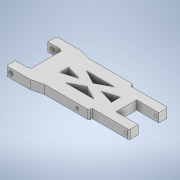
# Autodesk Inventor part: PX9200-10
Saved by Autodesk Inventor 2022.3 (Build 263350000, 350)
## iProperties
Created: 2022-07-14
Part Number: PX9200-10
Material: Generic
Document SubType Name: Modeling
Designer: luis_
Density: 1 g/cm^3
Appearance: Default
Author: luis_
Autodesk Inventor part; units mm, degrees
ref_plane "YZ Plane" through (0, 0, 0) normal (1, 0, 0) x (0, 1, 0)
ref_plane "XZ Plane" through (0, 0, 0) normal (0, 1, 0) x (-1, 0, 0)
ref_plane "XY Plane" through (0, 0, 0) normal (0, 0, 1) x (1, 0, 0)
sketch "Sketch1" plane through (0, 0, 0) normal (0, 1, 0) x (-1, 0, 0)
  line L0 (39.5, 16.9949) -> (118.5, 16.9949) construction
  line L1 (31.5, 10.9949) -> (39.5, 10.9949)
  line L2 (39.5, -11.0051) -> (31.5, -11.0051)
  line L3 (29.5, -10.0051) -> (31.5, -11.0051)
  line L4 (29.5, 9.9949) -> (31.5, 10.9949)
  line L5 (29.5, 9.9949) -> (29.5, -10.0051)
  line L6 (39.5, -17.0051) -> (39.5, -11.0051)
  line L7 (39.5, 10.9949) -> (39.5, 16.9949)
  line L8 (-14.5, 15) -> (15.5, 15)
  line L9 (15.5, -15) -> (-14.5, -15)
  line L10 (15.5, 15) -> (23.5, 16.9949)
  line L11 (15.5, -15) -> (23.5, -17.0051)
  line L12 (39.5, -17.0051) -> (23.5, -17.0051)
  line L13 (39.5, 16.9949) -> (23.5, 16.9949)
  line L14 (-39.5, 13) -> (-14.5, 13)
  line L15 (-39.5, -13) -> (-14.5, -13)
  line L16 (-24.5, 7) -> (-24.5, -7)
  line L17 (-24.5, 7) -> (-39.5, 7)
  line L18 (-24.5, -7) -> (-39.5, -7)
  line L19 (-39.5, 13) -> (-39.5, 7)
  line L20 (-39.5, -7) -> (-39.5, -13)
  line L21 (-17.5, 3) -> (-17.5, -3)
  line L22 (-17.5, 3) -> (-7.5, 0)
  line L23 (-7.5, 0) -> (-17.5, -3)
  line L24 (-14.5, 15) -> (-14.5, 13)
  line L25 (-14.5, -13) -> (-14.5, -15)
  line L26 (17.5, -3.0294) -> (17.5, 2.9706)
  line L27 (17.5, -3.0294) -> (7.5, -0.0294)
  line L28 (7.5, -0.0294) -> (17.5, 2.9706)
  line L29 (9.5, 7) -> (-9.5, 7)
  line L30 (0, 2) -> (9.5, 7)
  line L31 (-9.5, 7) -> (0, 2)
  line L32 (-9.5209, -7) -> (9.4791, -7)
  line L33 (-0.0209, -2) -> (-9.5209, -7)
  line L34 (9.4791, -7) -> (-0.0209, -2)
  point P0 (0, 0)
  point P1 (39.5, 13.9949)
  point P2 (-17.5, 0)
  point P3 (17.5, -0.0294)
  point P4 (-14.7945, 6.659)
  point P5 (-14.2279, -6.5477)
  point P6 (0, 7)
  point P7 (0, 7)
  dimension "d18" = 10
  dimension "d21" = 6
  dimension "d22" = 6
  dimension "d26" = 7
  dimension "d27" = 10
  dimension "d28" = 3
  dimension "d29" = 3
  dimension "d30" = 10
  dimension "d31" = 3
  dimension "d32" = 3
  constraints: 70 end point, 16 perpendicular, 5 parallel, 4 horizontal, 4 midpoint, 2 point on line, 1 coincident
  measures "d18" distance from line of L5 point (39.5, 13.995)
  measures "d21" distance between parallel lines of L14 L17
  measures "d22" distance between parallel lines of L15 L18
  measures "d26" distance between parallel lines of L16 L21
  measures "d27" distance from line of L21 L22.end
  measures "d28" distance of L21.end point (-17.5, 0)
  measures "d29" distance of L21.start point (-17.5, 0)
  measures "d30" distance from line of L26 L28.start
  measures "d31" distance of L26.end point (17.5, -0.029)
  measures "d32" distance of L26.start point (17.5, -0.029)
extrude "Extrusion1" add sketch "Sketch1" along normal blind 6
sketch "Sketch2" plane through (14.5, 0, 13) normal (0, 0, 1) x (1, 0, 0)
  line L0 (0, 6) -> (25, 6) projected
  line L1 (25, 0) -> (25, 6) projected
  circle A0 centre (23, 3) radius 1
  point P0 (-14.5, 0)
  point P1 (25, 3)
  dimension "d45" = 2
  constraints: 1 centre point, 1 midpoint
  measures "d45" diameter of A0
extrude "Extrusion2" cut sketch "Sketch2" against normal blind 40
sketch "Sketch3" plane through (-39.5, 0, 16.9949) normal (0, 0, 1) x (1, 0, 0)
  line L0 (8, 6) -> (0, 6) projected
  line L1 (0, 0) -> (0, 6) projected
  circle A0 centre (3.1, 3) radius 1.5
  point P0 (39.5, 0)
  dimension "d49" = 3
  constraints: 1 centre point
  measures "d49" diameter of A0
extrude "Extrusion3" cut sketch "Sketch3" against normal blind 40
fillet "Fillet1" radius 1 6 edges at (39.5, 3, -13) (14.5, 3, -15) (-39.5, 3, -17.0051) (39.5, 3, 13) (14.5, 3, 15) (-39.5, 3, 16.9949)
sketch "Sketch4" plane through (-15.5, 0, 15) normal (0, 0, 1) x (1, 0, 0)
  line L0 (-24, 0) -> (-24, 6)
  circle A0 centre (22, 3) radius 1
  point P0 (15.5, 0)
  dimension "d56" = 2
  constraints: 2 end point, 1 centre point, 1 coincident
  measures "d56" diameter of A0
extrude "Extrusion4" cut sketch "Sketch4" against normal blind 8
body "Solid1"
